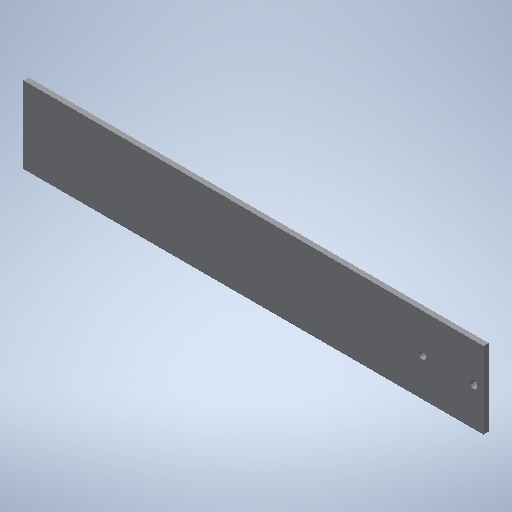
# Autodesk Inventor part: 海绵板
Saved by Autodesk Inventor 2025 (Build 290162000, 162)
## iProperties
Created: 2024-03-26
Part Number: 海绵板
Material: 常规
Document SubType Name: Modeling
Designer: Administrator
Density: 1 g/cm^3
Appearance: 默认
Author: Administrator
Autodesk Inventor part; units mm, degrees
ref_plane "YZ Plane" through (0, 0, 0) normal (1, 0, 0) x (0, 1, 0)
ref_plane "XZ Plane" through (0, 0, 0) normal (0, 1, 0) x (-1, 0, 0)
ref_plane "XY Plane" through (0, 0, 0) normal (0, 0, 1) x (1, 0, 0)
sketch "草图1" plane through (0, 0, 0) normal (0, 1, 0) x (-1, 0, 0)
  line L0 (-58.0948, -15) -> (-118.0948, -15)
  line L1 (-118.0948, -15) -> (-118.0948, 15)
  line L2 (-118.0948, 15) -> (-58.0948, 15)
  circle A0 centre (-94.0948, 0) radius 1.5
  circle A1 centre (-114.0948, 0) radius 1.5
  line L3 (-58.0948, 15) -> (61.9052, 15)
  line L4 (61.9052, 15) -> (61.9052, -15)
  line L5 (61.9052, -15) -> (-58.0948, -15)
  point P0 (0, 0)
  dimension "d12" = 30
  dimension "d15" = 3
  dimension "d16" = 3
  dimension "d19" = 180
  constraints: 12 end point, 3 perpendicular, 2 centre point, 1 horizontal, 1 parallel
  measures "d12" distance of L0.end L1.end
  measures "d15" diameter of A0
  measures "d16" diameter of A1
  measures "d19" distance of L1.end L3.end
extrude "拉伸2" add sketch "草图1" along normal blind 2
